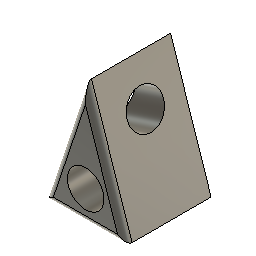
book_mark (Autodesk Fusion 360 design; units mm, degrees)
Autodesk Fusion 360 part; units mm, degrees
sketch "Sketch1" plane through (0, 0, 0) normal (0, 0, 1) x (1, 0, 0)
  line L0 (-25, 25) -> (25, 25)
  line L1 (25, 25) -> (25, -25)
  line L2 (25, -25) -> (-25, -25)
  line L3 (-25, -25) -> (-25, 25)
  constraint horizontal L0
  constraint vertical L1
  constraint horizontal L2
  constraint vertical L3
extrude "Extrude1" add sketch "Sketch1" along normal blind 75
sketch "Sketch2" plane through (0, -25, 0) normal (0, -1, 0) x (1, 0, 0)
  line L0 (-25, 0) -> (25, 0)
  line L1 (25, 0) -> (25, 75)
  line L2 (25, 75) -> (-25, 75)
  line L3 (-25, 75) -> (-25, 0)
  line L4 (-25, 0) -> (0, 75)
  line L5 (25, 0) -> (0, 75)
  line L6 (-25, 0) -> (25, 0)
  constraint coincident L0.start L3.end
  constraint midpoint L2 L4.end
  constraint coincident L0.end L1.start
extrude "Extrude2" add sketch "Sketch2" along normal blind 20 contours L0 L4 L5 L6
extrude "Extrude3" cut 1 faces at (16.6667, -25, 50) along direction (0, 1, 0) blind 95
extrude "Extrude4" cut 1 faces at (-16.6667, -25, 50) along direction (0, 1, 0) blind 65
move_face "OffsetFaces1" offset 50 1 faces at (-8.3333, 1.6667, 0)
extrude "Extrude5" cut 1 faces at (-13.8889, 1.6667, -50) along direction (0, 0, 1) blind 25
fillet "Fillet1" radius 5 1 faces at (0, -45, 8.3333)
hole "Hole1" at (0.1922, -45, -0.6545) direction (0, 1, 0) diameter 30 depth 100 tip angle 118
hole "Hole2" at (10.9055, -6.6558, 42.2834) direction (-0.948683, 0, -0.316228) diameter 30 depth 40 tip angle 118
